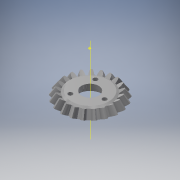
# Autodesk Inventor part: Kegelrad2
Saved by Autodesk Inventor 2018 (Build 220112000, 112)
## iProperties
Created: 2017-09-25
Part Number: Kegelrad2
Material: Steel, Mild
Document SubType Name: Modeling
Designer: JochenAlt
Categories: <?xml version="1.0" encoding="UTF-16"?> <MemberInstance><Categories><FamilyTemplate><FamilyTemplateParameter ValueType="xs:double" Id="1" ObjectReferenceKey="da_z" ObjectType="kUserParameterObject"/><FamilyTemplateParameter ValueType="xs:double" Id="2" ObjectReferenceKey="da_b" ObjectType="kUserParameterObject"/><FamilyTemplateParameter ValueType="xs:double" Id="3" ObjectReferenceKey="da_beta" ObjectType="kUserParameterObject"/><FamilyTemplateParameter ValueType="xs:double" Id="4" ObjectReferenceKey="da_dae" ObjectType="kUserParameterObject"/><FamilyTemplateParameter ValueType="xs:double" Id="5" ObjectReferenceKey="da_ve" ObjectType="kUserParameterObject"/><FamilyTemplateParameter ValueType="xs:double" Id="6" ObjectReferenceKey="da_omega" ObjectType="kUserParameterObject"/><FamilyTemplateParameter ValueType="xs:string" Id="7" ObjectReferenceKey="EAIAABAAAAAAHwAAAAAAAIAAAAAAAAAA" ObjectType="83914240" SubObjectId="SurfaceGeometry"/></FamilyTemplate><ParamToTemplateMap><ParamToTemplate CategoryParameter="//CategoryParameter[@InternalName='046C89C9-8512-4d59-83FE-43B91F4F132A']" TemplateParameter="1"/><ParamToTemplate CategoryParameter="//CategoryParameter[@InternalName='2552DF32-E462-4b46-AEBF-C6C7768E72AC']" TemplateParameter="2"/><ParamToTemplate CategoryParameter="//CategoryParameter[@InternalName='C9EE641D-15FC-4fae-A226-E94C4372FDD7']" TemplateParameter="3"/><ParamToTemplate><ParamToTemplate CategoryParameter="//CategoryParameter[@InternalName='00B6519A-459B-49c7-AD84-2E56D39A5744']" ConstantValue="-0.000000"/></ParamToTemplate><ParamToTemplate><ParamToTemplate CategoryParameter="//CategoryParameter[@InternalName='04B31F0E-C7A6-4894-AA32-9629BEFACF47']" ConstantValue="1.000000"/></ParamToTemplate><ParamToTemplate><ParamToTemplate CategoryParameter="//CategoryParameter[@InternalName='43CBEC2E-7847-49e7-A936-2F7889FCB2D9']" ConstantValue="0.200000"/></ParamToTemplate><ParamToTemplate><ParamToTemplate CategoryParameter="//CategoryParameter[@InternalName='B1EFC894-105D-4ebd-86BF-FA20ED196853']" ConstantValue="0.300000"/></ParamToTemplate><ParamToTemplate><ParamToTemplate CategoryParameter="//CategoryParameter[@InternalName='51175063-3D10-4879-93E8-6246FE8B403D']" ConstantValue="2060000000.000000"/></ParamToTemplate><ParamToTemplate><ParamToTemplate CategoryParameter="//CategoryParameter[@InternalName='A3A52E27-4454-46a9-B0BD-C932399B70AF']" ConstantValue="0.300000"/></ParamToTemplate><ParamToTemplate CategoryParameter="//CategoryParameter[@InternalName='2A200944-5A8C-41ca-B96E-8520D2E510F1']" TemplateParameter="4"/><ParamToTemplate><ParamToTemplate CategoryParameter="//CategoryParameter[@InternalName='1A637F62-92C8-44bc-B81F-10802510B579']" ConstantValue="2.383241"/></ParamToTemplate><ParamToTemplate CategoryParameter="//CategoryParameter[@InternalName='B52DD4BE-6863-48fb-BF58-89EF6F9EC65C']" TemplateParameter="5"/><ParamToTemplate><ParamToTemplate CategoryParameter="//CategoryParameter[@InternalName='3956BFF2-84D2-457d-93C2-9B0613DEBA67']" ConstantValue="1.729514"/></ParamToTemplate><ParamToTemplate CategoryParameter="//CategoryParameter[@InternalName='739CFA02-461B-4bf8-8049-181FCAD8B28F']" TemplateParameter="6"/><ParamToTemplate><ParamToTemplate CategoryParameter="//CategoryParameter[@InternalName='A27E999F-E2CE-4481-8A2A-EBF499C4C3C5']" ConstantValue="-0.000000"/></ParamToTemplate><ParamToTemplate><ParamToTemplate CategoryParameter="//CategoryParameter[@InternalName='9E1B4470-B2D3-4ff1-B813-535BB4CDF51A']" ConstantValue="3520000.000000"/></ParamToTemplate><ParamToTemplate><ParamToTemplate CategoryParameter="//CategoryParameter[@InternalName='F8452263-BFF6-458c-9FB1-07C4B99E95CD']" ConstantValue="11400000.000000"/></ParamToTemplate><ParamToTemplate><ParamToTemplate CategoryParameter="//CategoryParameter[@InternalName='3E3BB259-FD49-497f-8171-6EBC954A3479']" ConstantValue="2.000000"/></ParamToTemplate><ParamToTemplate CategoryParameter="//CategoryParameter[@InternalName='27C3BAF2-7550-4e4b-AE2C-0DB134B7D9B7']" TemplateParameter="7"/></ParamToTemplateMap><Category DisplayName="Gear" InternalName="DC85795E-93AB-48d5-8EEE-5A27447B64BD" Mnemonic="Gear"><CategoryParameter DisplayName="z" InternalName="046C89C9-8512-4d59-83FE-43B91F4F132A" Mnemonic="z"/><CategoryParameter DisplayName="b" InternalName="2552DF32-E462-4b46-AEBF-C6C7768E72AC" Mnemonic="b"/><CategoryParameter DisplayName="||b|" InternalName="C9EE641D-15FC-4fae-A226-E94C4372FDD7" Mnemonic="beta"/><CategoryParameter DisplayName="x" InternalName="00B6519A-459B-49c7-AD84-2E56D39A5744" Mnemonic="x"/><CategoryParameter DisplayName="a*" InternalName="04B31F0E-C7A6-4894-AA32-9629BEFACF47" Mnemonic="a"/><CategoryParameter DisplayName="c*" InternalName="43CBEC2E-7847-49e7-A936-2F7889FCB2D9" Mnemonic="c"/><CategoryParameter DisplayName="r|.f|*" InternalName="B1EFC894-105D-4ebd-86BF-FA20ED196853" Mnemonic="rf"/><CategoryParameter DisplayName="E" InternalName="51175063-3D10-4879-93E8-6246FE8B403D" Mnemonic="E"/><CategoryParameter DisplayName="||m|" InternalName="A3A52E27-4454-46a9-B0BD-C932399B70AF" Mnemonic="mi"/><Category DisplayName="BevelGear" InternalName="0C98F69A-0C2B-4791-B2FE-7691BB227E77" Mnemonic="BevelGear"><CategoryParameter DisplayName="d|.ae|" InternalName="2A200944-5A8C-41ca-B96E-8520D2E510F1" Mnemonic="dae"/><CategoryParameter DisplayName="d|.ai|" InternalName="1A637F62-92C8-44bc-B81F-10802510B579" Mnemonic="dai"/><CategoryParameter DisplayName="A|.e|" InternalName="B52DD4BE-6863-48fb-BF58-89EF6F9EC65C" Mnemonic="ve"/><CategoryParameter DisplayName="A|.i|" InternalName="3956BFF2-84D2-457d-93C2-9B0613DEBA67" Mnemonic="vi"/><CategoryParameter DisplayName="||S|" InternalName="739CFA02-461B-4bf8-8049-181FCAD8B28F" Mnemonic="omega"/><CategoryParameter DisplayName="x|.t|" InternalName="A27E999F-E2CE-4481-8A2A-EBF499C4C3C5" Mnemonic="xt"/><CategoryParameter DisplayName="||s||.Flim|" InternalName="9E1B4470-B2D3-4ff1-B813-535BB4CDF51A" Mnemonic="sFlim"/><CategoryParameter DisplayName="||s||.Hlim|" InternalName="F8452263-BFF6-458c-9FB1-07C4B99E95CD" Mnemonic="sHlim"/><CategoryParameter DisplayName="Typ" InternalName="3E3BB259-FD49-497f-8171-6EBC954A3479" Mnemonic="type"/><CategoryParameter DisplayName="PitchDiameter" InternalName="27C3BAF2-7550-4e4b-AE2C-0DB134B7D9B7" Mnemonic="IDS_PITCHDIAM"/></Category></Category></Categories></MemberInstance>
Mass: 60.9118 g
Surface Area: 34.3074 cm^2
Volume: 7.7496 cm^3
Density: 7.86 g/cm^3
Appearance: Steel
CustomPartVersion: 1
Author: JochenAlt
Autodesk Inventor part; units mm, degrees
ref_plane "XZ Plane" through (0, 0, 0) normal (0, 1, 0) x (-1, 0, 0)
ref_plane "Netzebene2" through (0, 0, 0) normal (0.9888308, 0.1490423, 0) x (0, 0, 1)
sketch "Skizze des Zahnradkörpers" plane through (0, 0, 0) normal (1, 0, 0) x (0, 1, 0)
  line L0 (0, 0) -> (11.8488, -22.0382) construction
  line L1 (11.8488, -22.0382) -> (14.1885, -20.5931)
  line L2 (14.1885, -20.5931) -> (0, 0) construction
  line L3 (13.125, -21.25) -> (0, 0) construction
  line L4 (9.9512, -18.5088) -> (11.9162, -17.2951)
  line L5 (11.8488, -22.0382) -> (9.9512, -18.5088)
  line L6 (14.1885, -20.5931) -> (11.9162, -17.2951)
  line L7 (0, -26.4126) -> (0, 4.4021) projected
  line L8 (0, -21.25) -> (14.1885, -21.25) construction
  dimension "d0" = 26.25
  dimension "d1" = 23.6976
  dimension "d2" = 28.377
  dimension "d3" = 4
  dimension "d4" = 20.5931
  constraints: 16 end point, 4 point on line, 3 perpendicular, 2 collinear, 1 horizontal alignment, 1 vertical alignment
  measures "d0" diameter of L3.start L7
  measures "d1" diameter of L0.end L7
  measures "d2" diameter of L1.end L7
  measures "d3" distance between parallel lines of L1 L4
  measures "d4" vertical distance of L1.end L0.start
revolve "Zahnradkörper" add sketch "Skizze des Zahnradkörpers" angle 360 about axis through (0, 0, 0) along (0, 0, 1)
ref_plane "Zahnebene" through (0, 13.125, -21.25) normal (0, -0.5254929, 0.850798) x (1, 0, 0)
sketch "Startskizze" plane through (0, 13.125, -21.25) normal (0, -0.5254929, 0.850798) x (1, 0, 0)
  line L0 (0, -17.8202) -> (0, 5.4053) projected
  arc A0 (-0.5181, -1.83) -> (-2.4185, 1.9071) centre (-6.193, -2.3641) ccw
  arc A1 (2.4185, 1.9071) -> (0.5181, -1.83) centre (6.193, -2.3641) ccw
  line L1 (-0.5181, -1.83) -> (0.5181, -1.83)
  arc A2 (2.4185, 1.9071) -> (-2.4185, 1.9071) centre (0, -15.4267) ccw
  dimension "d7" = 5.6999
  dimension "d8" = 6.193
  dimension "d9" = 13.0626
  dimension "d57" = 17.5017
  dimension "d58" = 13.5967
  constraints: 6 point on circle, 3 centre point, 3 symmetric about line, 2 end point, 1 coincident, 1 perpendicular, 1 other
  measures "d7" radius of A0
  measures "d8" horizontal distance of point (0, -15.427) A0.centre
  measures "d9" vertical distance of point (0, -15.427) A0.centre
  measures "d57" radius of A2
  measures "d58" distance from line of A2.centre L1
ref_plane "Endebene" through (0, 10.9508, -17.7298) normal (0, -0.5254929, 0.850798) x (1, 0, 0)
sketch "Endskizze" plane through (0, 10.9508, -17.7298) normal (0, -0.5254929, 0.850798) x (1, 0, 0)
  line L0 (0, -14.8329) -> (0, 4.518) projected
  arc A0 (-0.4328, -1.5133) -> (-2.0203, 1.6085) centre (-5.1733, -1.9594) ccw
  arc A1 (2.0203, 1.6085) -> (0.4328, -1.5133) centre (5.1733, -1.9594) ccw
  line L1 (-0.4328, -1.5133) -> (0.4328, -1.5133)
  arc A2 (2.0203, 1.6085) -> (-2.0203, 1.6085) centre (0, -12.8712) ccw
  dimension "d12" = 4.7614
  dimension "d15" = 5.1733
  dimension "d16" = 10.9118
  dimension "d59" = 14.6199
  dimension "d60" = 11.3579
  constraints: 6 point on circle, 3 centre point, 3 symmetric about line, 2 end point, 1 coincident, 1 other
  measures "d12" radius of A0
  measures "d15" horizontal distance of A0.centre point (0, -12.871)
  measures "d16" vertical distance of A0.centre point (0, -12.871)
  measures "d59" radius of A2
  measures "d60" distance from line of A2.centre L1
loft "Loft" cut profiles "Startskizze", "Endskizze"
pattern_circular "Circular Pattern" count 21 over 360 about axis through (0, 0, 0) along (0, 0, 1) of "Loft"
sketch3d "3D-Skizze rechts"
ref_plane "Endebene rechts" through (-0.8692, 10.9162, -17.7298) normal (0.041711, -0.5238349, 0.850798) x (0.9968448, 0.079375, 0)
sketch "Endskizze rechts" plane through (-0.8692, 10.9162, -17.7298) normal (0.041711, -0.5238349, 0.850798) x (0.9968448, 0.079375, 0)
  arc A0 (-0.4328, -1.5133) -> (-2.0203, 1.6085) centre (-5.1733, -1.9594) ccw
  line L0 (0, -16.7213) -> (0, 5.6038) projected
  arc A1 (2.0203, 1.6085) -> (0.4328, -1.5133) centre (5.1733, -1.9594) ccw
  line L1 (-0.4328, -1.5133) -> (0.4328, -1.5133)
  arc A2 (2.0203, 1.6085) -> (-2.0203, 1.6085) centre (0, -12.8712) ccw
  dimension "d70" = 5.1733
  dimension "d71" = 10.9118
  dimension "d72" = 4.7614
  dimension "d73" = 11.3579
  dimension "d74" = 14.6199
  constraints: 6 point on circle, 3 centre point, 3 symmetric about line, 2 end point, 1 coincident, 1 perpendicular, 1 other
  measures "d70" horizontal distance of A2.centre A0.centre
  measures "d71" vertical distance of point (0, -12.871) A0.centre
  measures "d72" radius of A0
  measures "d73" distance from line of point (0, -12.871) L1
  measures "d74" radius of A2
feature "Erhebung rechts" [suppressed]
pattern_circular "Runde Anordnung rechts" [suppressed]
sketch3d "3D-Skizze links"
ref_plane "Endebene links" through (0.863, 10.9162, -17.7283) normal (-0.0414159, -0.523874, 0.8507883) x (0.9968896, -0.0788111, 0)
sketch "Endskizze links" plane through (0.863, 10.9162, -17.7283) normal (-0.0414159, -0.523874, 0.8507883) x (0.9968896, -0.0788111, 0)
  line L0 (0, -24.7529) -> (0, 7.945) projected
  arc A0 (-0.4328, -1.5136) -> (-2.0203, 1.6081) centre (-5.1733, -1.9598) ccw
  arc A1 (2.0203, 1.6081) -> (0.4328, -1.5136) centre (5.1733, -1.9598) ccw
  line L1 (-0.4328, -1.5136) -> (0.4328, -1.5136)
  ellipse E0 centre (0, -9.0887) end of major axis (11.9162, -9.0887) minor radius 10.1382 projected
  arc A2 (2.0203, 1.6081) -> (-2.0203, 1.6081) centre (0, -12.8716) ccw
  dimension "d56" = 10.1382
  dimension "d30" = 4.7614
  dimension "d31" = 5.1733
  dimension "d32" = 10.9118
  dimension "d61" = 14.6199
  dimension "d62" = 11.3579
  constraints: 6 point on circle, 3 centre point, 3 symmetric about line, 2 end point, 1 coincident, 2 other
  measures "d30" radius of A0
  measures "d31" horizontal distance of point (0, -12.872) A0.centre
  measures "d32" vertical distance of A0.centre point (0, -12.872)
  measures "d61" radius of A2
  measures "d62" distance from line of point (0, -12.872) L1
feature "Erhebung links" [suppressed]
pattern_circular "Runde Anordnung links" [suppressed]
sketch "Körperskizze" plane through (0, 0, 0) normal (1, 0, 0) x (0, 1, 0)
  line L0 (0, -22.7248) -> (0, -17.7252) projected
  line L1 (11.8488, -22.0382) -> (9.9512, -18.5088) projected
  line L2 (9.9512, -18.5088) -> (0, -18.5088)
  line L3 (11.8488, -22.0382) -> (0, -22.0382)
  constraints: 4 end point, 2 perpendicular, 2 point on line
revolve "Festkörper" add sketch "Körperskizze" angle 360 about axis through (0, 0, 0) along (0, 0, 1)
sketch "Sketch6" plane through (0, 0, 0) normal (1, 0, 0) x (0, 1, 0)
  line L0 (13.125, -21.25) -> (0, 0) projected
  line L1 (0, -25.5) -> (0, 4.25) projected
surface revolve "Flankendurchmesser" sketch "Sketch6" angle 360 about axis through (0, 0, 0) along (0, 0, 1) shown no curves L0
sketch "Skizze9" plane through (0, 0, -18.5088) normal (0, 0, 1) x (1, 0, 0)
  circle A0 centre (0, 0) radius 9
  dimension "d109" = 18
  constraints: 1 centre point, 1 coincident
  measures "d109" diameter of A0
extrude "Extrusion4" add sketch "Skizze9" along normal blind 0.5
sketch "Skizze8" plane through (0, 0, -22.0382) normal (0, 0, -1) x (-1, 0, 0)
  circle A0 centre (-7, 0) radius 1.05
  circle A1 centre (3.5, 6.0622) radius 1.05
  circle A2 centre (3.5, -6.0622) radius 1.05
  circle A3 centre (0, 0) radius 5.6
  circle A4 centre (0, 0) radius 4.15
  dimension "d95" = 2.1
  dimension "d96" = 7
  dimension "d99" = 360
  dimension "d103" = 11.2
  dimension "d106" = 8.3
  constraints: 5 centre point, 2 coincident, 7 other
  measures "d95" diameter of A0
  measures "d96" distance of A0.centre point (0, 0)
  measures "d103" diameter of A3
  measures "d106" diameter of A4
extrude "Extrusion1" cut sketch "Skizze8" against normal up to next contours A0 | A1 | A2
extrude "Extrusion2" cut sketch "Skizze8" against normal blind 2.2 contours A3 | A4
extrude "Extrusion3" cut sketch "Skizze8" against normal through all contours A4
chamfer "Fase1" distance 0.951 distance2 0.5 1 edges at (-9, 0, -18.5088) measured on face at (-9.5, 0, -18.5088)
equation "\"d0\" = da_de"
equation "\"d1\" = da_dfe"
equation "\"d2\" = da_dae"
equation "\"d3\" = da_b"
equation "\"d4\" = da_ve"
equation "\"d7\" = fd_rr"
equation "\"d8\" = fd_x"
equation "\"d9\" = fd_y"
equation "\"d57\" = 0.5 * fd_dva + 0.3 * da_he"
equation "\"d58\" = 0.5 * fd_dva - 1.12 * da_he"
equation "\"da_teethtype\" = 0"
equation "\"d113\" = d110"
equation "\"da_b\" = 4"
equation "\"da_de\" = 26.25"
equation "\"da_dae\" = 28.37699"
equation "\"da_dfe\" = 23.69761"
equation "\"da_le\" = 24.97655"
equation "\"da_omega\" = 90deg"
equation "\"da_beta\" = 0"
equation "\"da_delta\" = 31.70143deg"
equation "\"da_alpha\" = 20deg"
equation "\"da_he\" = 2.75"
equation "\"da_ve\" = 20.59313"
equation "\"da_zv\" = 24.68271"
equation "\"fd_loft\" = da_b + 0.05 * da_he"
equation "\"fd_x\" = fd_x1 + fd_x2"
equation "\"fd_y\" = fd_y1 - fd_y2"
equation "\"fd_dd\" = fd_dva - 0.8 * da_he"
equation "\"da_dvw\" = 30.85339"
equation "\"d11\" = fd_loft"
equation "\"da_dm\" = 24.14803"
equation "\"da_x\" = 0"
equation "\"da_m\" = 1.25"
equation "\"d50\" = da_omega"
equation "\"fd_rr\" = 5.699931"
equation "\"fd_dva\" = 33.353387"
equation "\"d110\" = 0.5"
equation "\"fd_x1\" = 0.991971"
equation "\"fd_x2\" = 5.201001"
equation "\"fd_y1\" = 15.394768"
equation "\"fd_y2\" = 2.332125"
body "Solid1"
body "Srf1"
